Autodesk Fusion 360 part; units mm, degrees
(part 3 of 4)
  line L250 (188.6977, -24.525) -> (178.6977, -24.525)
  arc A251 (178.6977, -21.525) -> (178.6977, -24.525) centre (178.6977, -23.025) ccw
  line L251 (178.6977, -21.525) -> (188.6977, -21.525)
  arc A252 (188.6977, -34.525) -> (188.6977, -31.525) centre (188.6977, -33.025) ccw
  line L252 (188.6977, -34.525) -> (178.6977, -34.525)
  arc A253 (178.6977, -31.525) -> (178.6977, -34.525) centre (178.6977, -33.025) ccw
  line L253 (178.6977, -31.525) -> (188.6977, -31.525)
  arc A254 (88.6977, -34.525) -> (88.6977, -31.525) centre (88.6977, -33.025) ccw
  line L254 (88.6977, -34.525) -> (78.6977, -34.525)
  arc A255 (78.6977, -31.525) -> (78.6977, -34.525) centre (78.6977, -33.025) ccw
  line L255 (78.6977, -31.525) -> (88.6977, -31.525)
  arc A256 (228.6977, -64.525) -> (228.6977, -61.525) centre (228.6977, -63.025) ccw
  line L256 (228.6977, -64.525) -> (218.6977, -64.525)
  arc A257 (218.6977, -61.525) -> (218.6977, -64.525) centre (218.6977, -63.025) ccw
  line L257 (218.6977, -61.525) -> (228.6977, -61.525)
  arc A258 (148.6977, -14.525) -> (148.6977, -11.525) centre (148.6977, -13.025) ccw
  line L258 (148.6977, -14.525) -> (138.6977, -14.525)
  arc A259 (138.6977, -11.525) -> (138.6977, -14.525) centre (138.6977, -13.025) ccw
  line L259 (138.6977, -11.525) -> (148.6977, -11.525)
  arc A260 (208.6977, -54.525) -> (208.6977, -51.525) centre (208.6977, -53.025) ccw
  line L260 (208.6977, -54.525) -> (198.6977, -54.525)
  arc A261 (198.6977, -51.525) -> (198.6977, -54.525) centre (198.6977, -53.025) ccw
  line L261 (198.6977, -51.525) -> (208.6977, -51.525)
  arc A262 (148.6977, -44.525) -> (148.6977, -41.525) centre (148.6977, -43.025) ccw
  line L262 (148.6977, -44.525) -> (138.6977, -44.525)
  arc A263 (138.6977, -41.525) -> (138.6977, -44.525) centre (138.6977, -43.025) ccw
  line L263 (138.6977, -41.525) -> (148.6977, -41.525)
  arc A264 (108.6977, -54.525) -> (108.6977, -51.525) centre (108.6977, -53.025) ccw
  line L264 (108.6977, -54.525) -> (98.6977, -54.525)
  arc A265 (98.6977, -51.525) -> (98.6977, -54.525) centre (98.6977, -53.025) ccw
  line L265 (98.6977, -51.525) -> (108.6977, -51.525)
  arc A266 (108.6977, -24.525) -> (108.6977, -21.525) centre (108.6977, -23.025) ccw
  line L266 (108.6977, -24.525) -> (98.6977, -24.525)
  arc A267 (98.6977, -21.525) -> (98.6977, -24.525) centre (98.6977, -23.025) ccw
  line L267 (98.6977, -21.525) -> (108.6977, -21.525)
  arc A268 (168.6977, -44.525) -> (168.6977, -41.525) centre (168.6977, -43.025) ccw
  line L268 (168.6977, -44.525) -> (158.6977, -44.525)
  arc A269 (158.6977, -41.525) -> (158.6977, -44.525) centre (158.6977, -43.025) ccw
  line L269 (158.6977, -41.525) -> (168.6977, -41.525)
  arc A270 (168.6977, -54.525) -> (168.6977, -51.525) centre (168.6977, -53.025) ccw
  line L270 (168.6977, -54.525) -> (158.6977, -54.525)
  arc A271 (158.6977, -51.525) -> (158.6977, -54.525) centre (158.6977, -53.025) ccw
  line L271 (158.6977, -51.525) -> (168.6977, -51.525)
  arc A272 (148.6977, -34.525) -> (148.6977, -31.525) centre (148.6977, -33.025) ccw
  line L272 (148.6977, -34.525) -> (138.6977, -34.525)
  arc A273 (138.6977, -31.525) -> (138.6977, -34.525) centre (138.6977, -33.025) ccw
  line L273 (138.6977, -31.525) -> (148.6977, -31.525)
  arc A274 (228.6977, -34.525) -> (228.6977, -31.525) centre (228.6977, -33.025) ccw
  line L274 (228.6977, -34.525) -> (218.6977, -34.525)
  arc A275 (218.6977, -31.525) -> (218.6977, -34.525) centre (218.6977, -33.025) ccw
  line L275 (218.6977, -31.525) -> (228.6977, -31.525)
  arc A276 (128.6977, -14.525) -> (128.6977, -11.525) centre (128.6977, -13.025) ccw
  line L276 (128.6977, -14.525) -> (118.6977, -14.525)
  arc A277 (118.6977, -11.525) -> (118.6977, -14.525) centre (118.6977, -13.025) ccw
  line L277 (118.6977, -11.525) -> (128.6977, -11.525)
  arc A278 (108.6977, -44.525) -> (108.6977, -41.525) centre (108.6977, -43.025) ccw
  line L278 (108.6977, -44.525) -> (98.6977, -44.525)
  arc A279 (98.6977, -41.525) -> (98.6977, -44.525) centre (98.6977, -43.025) ccw
  line L279 (98.6977, -41.525) -> (108.6977, -41.525)
  arc A280 (248.6977, -54.525) -> (248.6977, -51.525) centre (248.6977, -53.025) ccw
  line L280 (248.6977, -54.525) -> (238.6977, -54.525)
  arc A281 (238.6977, -51.525) -> (238.6977, -54.525) centre (238.6977, -53.025) ccw
  line L281 (238.6977, -51.525) -> (248.6977, -51.525)
  arc A282 (128.6977, -24.525) -> (128.6977, -21.525) centre (128.6977, -23.025) ccw
  line L282 (128.6977, -24.525) -> (118.6977, -24.525)
  arc A283 (118.6977, -21.525) -> (118.6977, -24.525) centre (118.6977, -23.025) ccw
  line L283 (118.6977, -21.525) -> (128.6977, -21.525)
  arc A284 (108.6977, -34.525) -> (108.6977, -31.525) centre (108.6977, -33.025) ccw
  line L284 (108.6977, -34.525) -> (98.6977, -34.525)
  arc A285 (98.6977, -31.525) -> (98.6977, -34.525) centre (98.6977, -33.025) ccw
  line L285 (98.6977, -31.525) -> (108.6977, -31.525)
  arc A286 (148.6977, -24.525) -> (148.6977, -21.525) centre (148.6977, -23.025) ccw
  line L286 (148.6977, -24.525) -> (138.6977, -24.525)
  arc A287 (138.6977, -21.525) -> (138.6977, -24.525) centre (138.6977, -23.025) ccw
  line L287 (138.6977, -21.525) -> (148.6977, -21.525)
  arc A288 (148.6977, 35.475) -> (148.6977, 38.475) centre (148.6977, 36.975) ccw
  line L288 (148.6977, 35.475) -> (138.6977, 35.475)
  arc A289 (138.6977, 38.475) -> (138.6977, 35.475) centre (138.6977, 36.975) ccw
  line L289 (138.6977, 38.475) -> (148.6977, 38.475)
  arc A290 (208.6977, 15.475) -> (208.6977, 18.475) centre (208.6977, 16.975) ccw
  line L290 (208.6977, 15.475) -> (198.6977, 15.475)
  arc A291 (198.6977, 18.475) -> (198.6977, 15.475) centre (198.6977, 16.975) ccw
  line L291 (198.6977, 18.475) -> (208.6977, 18.475)
  arc A292 (148.6977, 5.475) -> (148.6977, 8.475) centre (148.6977, 6.975) ccw
  line L292 (148.6977, 5.475) -> (138.6977, 5.475)
  arc A293 (138.6977, 8.475) -> (138.6977, 5.475) centre (138.6977, 6.975) ccw
  line L293 (138.6977, 8.475) -> (148.6977, 8.475)
  arc A294 (228.6977, -4.525) -> (228.6977, -1.525) centre (228.6977, -3.025) ccw
  line L294 (228.6977, -4.525) -> (218.6977, -4.525)
  arc A295 (218.6977, -1.525) -> (218.6977, -4.525) centre (218.6977, -3.025) ccw
  line L295 (218.6977, -1.525) -> (228.6977, -1.525)
  arc A296 (188.6977, 15.475) -> (188.6977, 18.475) centre (188.6977, 16.975) ccw
  line L296 (188.6977, 15.475) -> (178.6977, 15.475)
  arc A297 (178.6977, 18.475) -> (178.6977, 15.475) centre (178.6977, 16.975) ccw
  line L297 (178.6977, 18.475) -> (188.6977, 18.475)
  arc A298 (208.6977, -4.525) -> (208.6977, -1.525) centre (208.6977, -3.025) ccw
  line L298 (208.6977, -4.525) -> (198.6977, -4.525)
  arc A299 (198.6977, -1.525) -> (198.6977, -4.525) centre (198.6977, -3.025) ccw
  line L299 (198.6977, -1.525) -> (208.6977, -1.525)
  arc A300 (148.6977, 15.475) -> (148.6977, 18.475) centre (148.6977, 16.975) ccw
  line L300 (148.6977, 15.475) -> (138.6977, 15.475)
  arc A301 (138.6977, 18.475) -> (138.6977, 15.475) centre (138.6977, 16.975) ccw
  line L301 (138.6977, 18.475) -> (148.6977, 18.475)
  arc A302 (188.6977, 25.475) -> (188.6977, 28.475) centre (188.6977, 26.975) ccw
  line L302 (188.6977, 25.475) -> (178.6977, 25.475)
  arc A303 (178.6977, 28.475) -> (178.6977, 25.475) centre (178.6977, 26.975) ccw
  line L303 (178.6977, 28.475) -> (188.6977, 28.475)
  arc A304 (128.6977, 5.475) -> (128.6977, 8.475) centre (128.6977, 6.975) ccw
  line L304 (128.6977, 5.475) -> (118.6977, 5.475)
  arc A305 (118.6977, 8.475) -> (118.6977, 5.475) centre (118.6977, 6.975) ccw
  line L305 (118.6977, 8.475) -> (128.6977, 8.475)
  arc A306 (168.6977, 25.475) -> (168.6977, 28.475) centre (168.6977, 26.975) ccw
  line L306 (168.6977, 25.475) -> (158.6977, 25.475)
  arc A307 (158.6977, 28.475) -> (158.6977, 25.475) centre (158.6977, 26.975) ccw
  line L307 (158.6977, 28.475) -> (168.6977, 28.475)
  arc A308 (168.6977, -4.525) -> (168.6977, -1.525) centre (168.6977, -3.025) ccw
  line L308 (168.6977, -4.525) -> (158.6977, -4.525)
  arc A309 (158.6977, -1.525) -> (158.6977, -4.525) centre (158.6977, -3.025) ccw
  line L309 (158.6977, -1.525) -> (168.6977, -1.525)
  arc A310 (208.6977, 25.475) -> (208.6977, 28.475) centre (208.6977, 26.975) ccw
  line L310 (208.6977, 25.475) -> (198.6977, 25.475)
  arc A311 (198.6977, 28.475) -> (198.6977, 25.475) centre (198.6977, 26.975) ccw
  line L311 (198.6977, 28.475) -> (208.6977, 28.475)
  arc A312 (168.6977, 35.475) -> (168.6977, 38.475) centre (168.6977, 36.975) ccw
  line L312 (168.6977, 35.475) -> (158.6977, 35.475)
  arc A313 (158.6977, 38.475) -> (158.6977, 35.475) centre (158.6977, 36.975) ccw
  line L313 (158.6977, 38.475) -> (168.6977, 38.475)
  arc A314 (228.6977, 15.475) -> (228.6977, 18.475) centre (228.6977, 16.975) ccw
  line L314 (228.6977, 15.475) -> (218.6977, 15.475)
  arc A315 (218.6977, 18.475) -> (218.6977, 15.475) centre (218.6977, 16.975) ccw
  line L315 (218.6977, 18.475) -> (228.6977, 18.475)
  arc A316 (168.6977, 15.475) -> (168.6977, 18.475) centre (168.6977, 16.975) ccw
  line L316 (168.6977, 15.475) -> (158.6977, 15.475)
  arc A317 (158.6977, 18.475) -> (158.6977, 15.475) centre (158.6977, 16.975) ccw
  line L317 (158.6977, 18.475) -> (168.6977, 18.475)
  arc A318 (188.6977, 5.475) -> (188.6977, 8.475) centre (188.6977, 6.975) ccw
  line L318 (188.6977, 5.475) -> (178.6977, 5.475)
  arc A319 (178.6977, 8.475) -> (178.6977, 5.475) centre (178.6977, 6.975) ccw
  line L319 (178.6977, 8.475) -> (188.6977, 8.475)
  arc A320 (148.6977, -4.525) -> (148.6977, -1.525) centre (148.6977, -3.025) ccw
  line L320 (148.6977, -4.525) -> (138.6977, -4.525)
  arc A321 (138.6977, -1.525) -> (138.6977, -4.525) centre (138.6977, -3.025) ccw
  line L321 (138.6977, -1.525) -> (148.6977, -1.525)
  arc A322 (208.6977, 5.475) -> (208.6977, 8.475) centre (208.6977, 6.975) ccw
  line L322 (208.6977, 5.475) -> (198.6977, 5.475)
  arc A323 (198.6977, 8.475) -> (198.6977, 5.475) centre (198.6977, 6.975) ccw
  line L323 (198.6977, 8.475) -> (208.6977, 8.475)
  arc A324 (168.6977, 5.475) -> (168.6977, 8.475) centre (168.6977, 6.975) ccw
  line L324 (168.6977, 5.475) -> (158.6977, 5.475)
  arc A325 (158.6977, 8.475) -> (158.6977, 5.475) centre (158.6977, 6.975) ccw
  line L325 (158.6977, 8.475) -> (168.6977, 8.475)
  arc A326 (228.6977, 5.475) -> (228.6977, 8.475) centre (228.6977, 6.975) ccw
  line L326 (228.6977, 5.475) -> (218.6977, 5.475)
  arc A327 (218.6977, 8.475) -> (218.6977, 5.475) centre (218.6977, 6.975) ccw
  line L327 (218.6977, 8.475) -> (228.6977, 8.475)
  arc A328 (188.6977, -4.525) -> (188.6977, -1.525) centre (188.6977, -3.025) ccw
  line L328 (188.6977, -4.525) -> (178.6977, -4.525)
  arc A329 (178.6977, -1.525) -> (178.6977, -4.525) centre (178.6977, -3.025) ccw
  line L329 (178.6977, -1.525) -> (188.6977, -1.525)
  arc A330 (148.6977, 25.475) -> (148.6977, 28.475) centre (148.6977, 26.975) ccw
  line L330 (148.6977, 25.475) -> (138.6977, 25.475)
  arc A331 (138.6977, 28.475) -> (138.6977, 25.475) centre (138.6977, 26.975) ccw
  line L331 (138.6977, 28.475) -> (148.6977, 28.475)
  arc A332 (188.6977, 35.475) -> (188.6977, 38.475) centre (188.6977, 36.975) ccw
  line L332 (188.6977, 35.475) -> (178.6977, 35.475)
  arc A333 (178.6977, 38.475) -> (178.6977, 35.475) centre (178.6977, 36.975) ccw
  line L333 (178.6977, 38.475) -> (188.6977, 38.475)
  arc A334 (208.6977, 35.475) -> (208.6977, 38.475) centre (208.6977, 36.975) ccw
  line L334 (208.6977, 35.475) -> (198.6977, 35.475)
  arc A335 (198.6977, 38.475) -> (198.6977, 35.475) centre (198.6977, 36.975) ccw
  line L335 (198.6977, 38.475) -> (208.6977, 38.475)
  line L336 (105.9194, -146.05) -> (128.4396, -191.0218)
  line L337 (128.4396, -191.0218) -> (228.4396, -191.0218)
  line L338 (228.4396, -191.0218) -> (250, -146.0218)
  line L339 (250, -146.0218) -> (269.4662, -146.0492)
  line L340 (269.4662, -146.0492) -> (269.5337, -0.009)
  line L341 (269.5337, -0.009) -> (249.9865, 0)
  line L342 (249.9865, 0) -> (228.4396, 44.9718)
  line L343 (228.4396, 44.9718) -> (128.4396, 44.9718)
  line L344 (128.4396, 44.9718) -> (105.9194, 0)
  line L345 (105.9194, 0) -> (90, 0)
  line L346 (90, 0) -> (60, -38.025)
  line L347 (60, -38.025) -> (17.3954, -46.901)
  line L348 (17.3954, -46.901) -> (17.3954, -99.149)
  line L349 (17.3954, -99.149) -> (60, -108.025)
  line L350 (60, -108.025) -> (90, -146.05)
  line L351 (90, -146.05) -> (105.9194, -146.05)
  line L352 (46.3999, -83.0262) -> (46.3999, -63.0262)
  line L353 (46.3999, -63.0262) -> (53.3999, -63.0262)
  line L354 (53.3999, -63.0262) -> (53.3999, -83.0262)
  line L355 (53.3999, -83.0262) -> (46.3999, -83.0262)
copy_body "Body->Comp1" bodies 1 removing the originals makes body 2 in component "Electronics Plate"
sketch "Sketch9" plane through (0, 5, 0) normal (0, 1, 0) x (-1, 0, 0)
  circle A0 centre (260, -3.75) radius 1.5
  circle A1 centre (245, -3.75) radius 1.5
  circle A2 centre (230, -3.75) radius 1.5
  line L0 (250, -73) -> (238, -73) construction
  line L1 (270, -146) -> (220, -146) construction
  line L2 (220, -146) -> (220, -138.5) construction
  line L3 (220, -138.5) -> (270, -138.5) construction
  line L4 (270, -138.5) -> (270, -146) construction
  circle A3 centre (260, -142.25) radius 1.5
  circle A4 centre (245, -142.25) radius 1.5
  circle A5 centre (230, -142.25) radius 1.5
  dimension "d102" = 3
  dimension "d103" = 3
  dimension "d104" = 3
  dimension "d106" = 15
  dimension "d107" = 15
  dimension "d108" = 50
  dimension "d109" = 7.5
  dimension "d110" = 3
  dimension "d111" = 3
  dimension "d112" = 3
  dimension "d113" = 10
  dimension "d114" = 15
  dimension "d115" = 15
  constraint horizontal L0
  constraint horizontal L1
  constraint vertical L2
  constraint horizontal L3
  constraint vertical L4
  measures "d102" diameter of A0
  measures "d103" diameter of A1
  measures "d104" diameter of A2
  measures "d106" distance of A0.centre A1.centre
  measures "d107" distance of A1.centre A2.centre
  measures "d108" distance of L1.start L1.end
  measures "d109" distance of L1.start L3.end
  measures "d110" diameter of A3
  measures "d111" diameter of A4
  measures "d112" diameter of A5
  measures "d113" distance of L4 A3.centre
  measures "d114" distance of A3.centre A4.centre
  measures "d115" distance of A4.centre A5.centre
extrude "Extrude1" cut sketch "Sketch9" against normal blind 40 bodies 2 in component "Electronics Plate"
fillet "Fillet1" radius 30 2 edges at (-90, 2.5, 0) (-90, 2.5, -146.05) on bodies 2 in component "Electronics Plate"
fillet "Fillet2" radius 5 4 edges at (-269.5337, 2.5, -0.009) (-269.4662, 2.5, -146.0492) (-17.3954, 2.5, -46.901) (-17.3954, 2.5, -99.149) on bodies 2 in component "Electronics Plate"
fillet "Fillet3" radius 20 2 edges at (-60, 2.5, -38.025) (-60, 2.5, -108.025) on bodies 2 in component "Electronics Plate"
fillet "Fillet4" radius 17.5 2 edges at (-105.9194, 2.5, 0) (-105.9194, 2.5, -146.05) on bodies 2 in component "Electronics Plate"
fillet "Fillet5" radius 10 4 edges at (-128.4396, 2.5, -191.0218) (-228.4396, 2.5, -191.0218) (-228.4396, 2.5, 44.9718) (-128.4396, 2.5, 44.9718) on bodies 2 in component "Electronics Plate"
sketch "Sketch10" plane through (0, 5, 0) normal (0, 1, 0) x (-1, 0, 0)
sketch "Sketch11" plane through (0, 5, 0) normal (0, 1, 0) x (-1, 0, 0)
  arc A0 (134.6157, 44.9718) -> (125.6742, 39.4494) centre (134.6157, 34.9718) ccw
  line L0 (125.6742, 39.4494) -> (110.2299, 8.6079)
  arc A1 (98.2523, -0.6672) -> (110.2299, 8.6079) centre (94.5822, 16.4437) ccw
  arc A2 (98.2523, -0.6672) -> (80.9916, -11.4182) centre (104.544, -30) ccw
  line L1 (80.9916, -11.4182) -> (64.5039, -32.3163)
  arc A3 (52.8814, -39.508) -> (64.5039, -32.3163) centre (48.8023, -19.9284) ccw
  line L2 (52.8814, -39.508) -> (21.3756, -46.0717)
  arc A4 (21.3756, -46.0717) -> (17.3954, -50.9667) centre (22.3954, -50.9667) ccw
  line L3 (17.3954, -50.9667) -> (17.3954, -95.0833)
  arc A5 (17.3954, -95.0833) -> (21.3756, -99.9783) centre (22.3954, -95.0833) ccw
  line L4 (21.3756, -99.9783) -> (52.8814, -106.542)
  arc A6 (64.5039, -113.7337) -> (52.8814, -106.542) centre (48.8023, -126.1216) ccw
  line L5 (64.5039, -113.7337) -> (80.9916, -134.6318)
  arc A7 (80.9916, -134.6318) -> (98.2523, -145.3828) centre (104.544, -116.05) ccw
  arc A8 (110.2299, -154.6579) -> (98.2523, -145.3828) centre (94.5822, -162.4937) ccw
  line L6 (110.2299, -154.6579) -> (125.6742, -185.4994)
  arc A9 (125.6742, -185.4994) -> (134.6157, -191.0218) centre (134.6157, -181.0218) ccw
  line L7 (134.6157, -191.0218) -> (222.1423, -191.0218)
  arc A10 (222.1423, -191.0218) -> (231.1606, -185.3427) centre (222.1423, -181.0218) ccw
  line L8 (231.1606, -185.3427) -> (250, -146.0218)
  line L9 (250, -146.0218) -> (264.4614, -146.0422)
  arc A11 (264.4614, -146.0422) -> (269.4685, -141.0445) centre (264.4685, -141.0422) ccw
  line L10 (269.4685, -141.0445) -> (269.5314, -5.009)
  arc A12 (269.5314, -5.009) -> (264.5337, -0.0067) centre (264.5314, -5.0067) ccw
  line L11 (264.5337, -0.0067) -> (249.9865, 0)
  line L12 (249.9865, 0) -> (231.1606, 39.2927)
  arc A13 (231.1606, 39.2927) -> (222.1423, 44.9718) centre (222.1423, 34.9718) ccw
  line L13 (222.1423, 44.9718) -> (134.6157, 44.9718)
  arc A14 (228.7157, -4.5249) -> (229.982, -2.2501) centre (230, -3.75) ccw
  arc A15 (228.6977, -4.525) -> (228.7157, -4.5249) centre (228.6977, -3.025) ccw
  line L14 (228.6977, -4.525) -> (218.6977, -4.525)
  arc A16 (218.6977, -1.525) -> (218.6977, -4.525) centre (218.6977, -3.025) ccw
  line L15 (218.6977, -1.525) -> (228.6977, -1.525)
  arc A17 (229.982, -2.2501) -> (228.6977, -1.525) centre (228.6977, -3.025) ccw
  circle A18 centre (260, -3.75) radius 1.5
  circle A19 centre (260, -142.25) radius 1.5
  circle A20 centre (245, -3.75) radius 1.5
  circle A21 centre (245, -142.25) radius 1.5
  arc A22 (208.6977, 15.475) -> (208.6977, 18.475) centre (208.6977, 16.975) ccw
  line L16 (208.6977, 15.475) -> (198.6977, 15.475)
  arc A23 (198.6977, 18.475) -> (198.6977, 15.475) centre (198.6977, 16.975) ccw
  line L17 (198.6977, 18.475) -> (208.6977, 18.475)
  arc A24 (108.6977, -34.525) -> (108.6977, -31.525) centre (108.6977, -33.025) ccw
  line L18 (108.6977, -34.525) -> (98.6977, -34.525)
  arc A25 (98.6977, -31.525) -> (98.6977, -34.525) centre (98.6977, -33.025) ccw
  line L19 (98.6977, -31.525) -> (108.6977, -31.525)
  arc A26 (88.6977, -44.525) -> (88.6977, -41.525) centre (88.6977, -43.025) ccw
  line L20 (88.6977, -44.525) -> (78.6977, -44.525)
  arc A27 (78.6977, -41.525) -> (78.6977, -44.525) centre (78.6977, -43.025) ccw
  line L21 (78.6977, -41.525) -> (88.6977, -41.525)
  arc A28 (168.6977, -34.525) -> (168.6977, -31.525) centre (168.6977, -33.025) ccw
  line L22 (168.6977, -34.525) -> (158.6977, -34.525)
  arc A29 (158.6977, -31.525) -> (158.6977, -34.525) centre (158.6977, -33.025) ccw
  line L23 (158.6977, -31.525) -> (168.6977, -31.525)
  arc A30 (148.6977, -44.525) -> (148.6977, -41.525) centre (148.6977, -43.025) ccw
  line L24 (148.6977, -44.525) -> (138.6977, -44.525)
  arc A31 (138.6977, -41.525) -> (138.6977, -44.525) centre (138.6977, -43.025) ccw
  line L25 (138.6977, -41.525) -> (148.6977, -41.525)
  arc A32 (168.6977, -24.525) -> (168.6977, -21.525) centre (168.6977, -23.025) ccw
  line L26 (168.6977, -24.525) -> (158.6977, -24.525)
  arc A33 (158.6977, -21.525) -> (158.6977, -24.525) centre (158.6977, -23.025) ccw
  line L27 (158.6977, -21.525) -> (168.6977, -21.525)
  arc A34 (228.6977, -34.525) -> (228.6977, -31.525) centre (228.6977, -33.025) ccw
  line L28 (228.6977, -34.525) -> (218.6977, -34.525)
  arc A35 (218.6977, -31.525) -> (218.6977, -34.525) centre (218.6977, -33.025) ccw
  line L29 (218.6977, -31.525) -> (228.6977, -31.525)
  arc A36 (148.6977, -34.525) -> (148.6977, -31.525) centre (148.6977, -33.025) ccw
  line L30 (148.6977, -34.525) -> (138.6977, -34.525)
  arc A37 (138.6977, -31.525) -> (138.6977, -34.525) centre (138.6977, -33.025) ccw
  line L31 (138.6977, -31.525) -> (148.6977, -31.525)
  arc A38 (148.6977, 5.475) -> (148.6977, 8.475) centre (148.6977, 6.975) ccw
  line L32 (148.6977, 5.475) -> (138.6977, 5.475)
  arc A39 (138.6977, 8.475) -> (138.6977, 5.475) centre (138.6977, 6.975) ccw
  line L33 (138.6977, 8.475) -> (148.6977, 8.475)
  arc A40 (168.6977, -4.525) -> (168.6977, -1.525) centre (168.6977, -3.025) ccw
  line L34 (168.6977, -4.525) -> (158.6977, -4.525)
  arc A41 (158.6977, -1.525) -> (158.6977, -4.525) centre (158.6977, -3.025) ccw
  line L35 (158.6977, -1.525) -> (168.6977, -1.525)
  arc A42 (228.6977, -14.525) -> (228.6977, -11.525) centre (228.6977, -13.025) ccw
  line L36 (228.6977, -14.525) -> (218.6977, -14.525)
  arc A43 (218.6977, -11.525) -> (218.6977, -14.525) centre (218.6977, -13.025) ccw
  line L37 (218.6977, -11.525) -> (228.6977, -11.525)
  arc A44 (168.6977, -14.525) -> (168.6977, -11.525) centre (168.6977, -13.025) ccw
  line L38 (168.6977, -14.525) -> (158.6977, -14.525)
  arc A45 (158.6977, -11.525) -> (158.6977, -14.525) centre (158.6977, -13.025) ccw
  line L39 (158.6977, -11.525) -> (168.6977, -11.525)
  arc A46 (188.6977, -34.525) -> (188.6977, -31.525) centre (188.6977, -33.025) ccw
  line L40 (188.6977, -34.525) -> (178.6977, -34.525)
  arc A47 (178.6977, -31.525) -> (178.6977, -34.525) centre (178.6977, -33.025) ccw
  line L41 (178.6977, -31.525) -> (188.6977, -31.525)
  arc A48 (148.6977, -4.525) -> (148.6977, -1.525) centre (148.6977, -3.025) ccw
  line L42 (148.6977, -4.525) -> (138.6977, -4.525)
  arc A49 (138.6977, -1.525) -> (138.6977, -4.525) centre (138.6977, -3.025) ccw
  line L43 (138.6977, -1.525) -> (148.6977, -1.525)
  arc A50 (108.6977, -14.525) -> (108.6977, -11.525) centre (108.6977, -13.025) ccw
  line L44 (108.6977, -14.525) -> (98.6977, -14.525)
  arc A51 (98.6977, -11.525) -> (98.6977, -14.525) centre (98.6977, -13.025) ccw
  line L45 (98.6977, -11.525) -> (108.6977, -11.525)
  arc A52 (248.6977, -24.525) -> (248.6977, -21.525) centre (248.6977, -23.025) ccw
  line L46 (248.6977, -24.525) -> (238.6977, -24.525)
  arc A53 (238.6977, -21.525) -> (238.6977, -24.525) centre (238.6977, -23.025) ccw
  line L47 (238.6977, -21.525) -> (248.6977, -21.525)
  arc A54 (148.6977, 35.475) -> (148.6977, 38.475) centre (148.6977, 36.975) ccw
  line L48 (148.6977, 35.475) -> (138.6977, 35.475)
  arc A55 (138.6977, 38.475) -> (138.6977, 35.475) centre (138.6977, 36.975) ccw
  line L49 (138.6977, 38.475) -> (148.6977, 38.475)
  arc A56 (128.6977, -4.525) -> (128.6977, -1.525) centre (128.6977, -3.025) ccw
  line L50 (128.6977, -4.525) -> (118.6977, -4.525)
  arc A57 (118.6977, -1.525) -> (118.6977, -4.525) centre (118.6977, -3.025) ccw
  line L51 (118.6977, -1.525) -> (128.6977, -1.525)
  arc A58 (168.6977, 35.475) -> (168.6977, 38.475) centre (168.6977, 36.975) ccw
  line L52 (168.6977, 35.475) -> (158.6977, 35.475)
  arc A59 (158.6977, 38.475) -> (158.6977, 35.475) centre (158.6977, 36.975) ccw
  line L53 (158.6977, 38.475) -> (168.6977, 38.475)
  arc A60 (168.6977, -44.525) -> (168.6977, -41.525) centre (168.6977, -43.025) ccw
  line L54 (168.6977, -44.525) -> (158.6977, -44.525)
  arc A61 (158.6977, -41.525) -> (158.6977, -44.525) centre (158.6977, -43.025) ccw
  line L55 (158.6977, -41.525) -> (168.6977, -41.525)
  arc A62 (248.6977, -54.525) -> (248.6977, -51.525) centre (248.6977, -53.025) ccw
  line L56 (248.6977, -54.525) -> (238.6977, -54.525)
  arc A63 (238.6977, -51.525) -> (238.6977, -54.525) centre (238.6977, -53.025) ccw
  line L57 (238.6977, -51.525) -> (248.6977, -51.525)
  arc A64 (128.6977, -24.525) -> (128.6977, -21.525) centre (128.6977, -23.025) ccw
  line L58 (128.6977, -24.525) -> (118.6977, -24.525)
  arc A65 (118.6977, -21.525) -> (118.6977, -24.525) centre (118.6977, -23.025) ccw
  line L59 (118.6977, -21.525) -> (128.6977, -21.525)
  arc A66 (188.6977, -24.525) -> (188.6977, -21.525) centre (188.6977, -23.025) ccw
  line L60 (188.6977, -24.525) -> (178.6977, -24.525)
  arc A67 (178.6977, -21.525) -> (178.6977, -24.525) centre (178.6977, -23.025) ccw
  line L61 (178.6977, -21.525) -> (188.6977, -21.525)
  arc A68 (228.6977, -44.525) -> (228.6977, -41.525) centre (228.6977, -43.025) ccw
  line L62 (228.6977, -44.525) -> (218.6977, -44.525)
  arc A69 (218.6977, -41.525) -> (218.6977, -44.525) centre (218.6977, -43.025) ccw
  line L63 (218.6977, -41.525) -> (228.6977, -41.525)
  arc A70 (188.6977, -44.525) -> (188.6977, -41.525) centre (188.6977, -43.025) ccw
  line L64 (188.6977, -44.525) -> (178.6977, -44.525)
  arc A71 (178.6977, -41.525) -> (178.6977, -44.525) centre (178.6977, -43.025) ccw
  line L65 (178.6977, -41.525) -> (188.6977, -41.525)
  arc A72 (228.6977, 15.475) -> (228.6977, 18.475) centre (228.6977, 16.975) ccw
  line L66 (228.6977, 15.475) -> (218.6977, 15.475)
  arc A73 (218.6977, 18.475) -> (218.6977, 15.475) centre (218.6977, 16.975) ccw
  line L67 (218.6977, 18.475) -> (228.6977, 18.475)
  arc A74 (148.6977, -74.525) -> (148.6977, -71.525) centre (148.6977, -73.025) ccw
  line L68 (148.6977, -74.525) -> (138.6977, -74.525)
  arc A75 (138.6977, -71.525) -> (138.6977, -74.525) centre (138.6977, -73.025) ccw
  line L69 (138.6977, -71.525) -> (148.6977, -71.525)
  arc A76 (228.6977, -24.525) -> (228.6977, -21.525) centre (228.6977, -23.025) ccw
  line L70 (228.6977, -24.525) -> (218.6977, -24.525)
  arc A77 (218.6977, -21.525) -> (218.6977, -24.525) centre (218.6977, -23.025) ccw
  line L71 (218.6977, -21.525) -> (228.6977, -21.525)
  arc A78 (248.6977, -34.525) -> (248.6977, -31.525) centre (248.6977, -33.025) ccw
  line L72 (248.6977, -34.525) -> (238.6977, -34.525)
  arc A79 (238.6977, -31.525) -> (238.6977, -34.525) centre (238.6977, -33.025) ccw
  line L73 (238.6977, -31.525) -> (248.6977, -31.525)
  arc A80 (128.6977, 5.475) -> (128.6977, 8.475) centre (128.6977, 6.975) ccw
  line L74 (128.6977, 5.475) -> (118.6977, 5.475)
  arc A81 (118.6977, 8.475) -> (118.6977, 5.475) centre (118.6977, 6.975) ccw
  line L75 (118.6977, 8.475) -> (128.6977, 8.475)
  arc A82 (228.6977, 5.475) -> (228.6977, 8.475) centre (228.6977, 6.975) ccw
  line L76 (228.6977, 5.475) -> (218.6977, 5.475)
  arc A83 (218.6977, 8.475) -> (218.6977, 5.475) centre (218.6977, 6.975) ccw
  line L77 (218.6977, 8.475) -> (228.6977, 8.475)
  arc A84 (208.6977, 25.475) -> (208.6977, 28.475) centre (208.6977, 26.975) ccw
  line L78 (208.6977, 25.475) -> (198.6977, 25.475)
  arc A85 (198.6977, 28.475) -> (198.6977, 25.475) centre (198.6977, 26.975) ccw
  line L79 (198.6977, 28.475) -> (208.6977, 28.475)
  arc A86 (148.6977, 15.475) -> (148.6977, 18.475) centre (148.6977, 16.975) ccw
  line L80 (148.6977, 15.475) -> (138.6977, 15.475)
  arc A87 (138.6977, 18.475) -> (138.6977, 15.475) centre (138.6977, 16.975) ccw
  line L81 (138.6977, 18.475) -> (148.6977, 18.475)
  arc A88 (108.6977, -44.525) -> (108.6977, -41.525) centre (108.6977, -43.025) ccw
  line L82 (108.6977, -44.525) -> (98.6977, -44.525)
  arc A89 (98.6977, -41.525) -> (98.6977, -44.525) centre (98.6977, -43.025) ccw
  line L83 (98.6977, -41.525) -> (108.6977, -41.525)
  arc A90 (168.6977, 25.475) -> (168.6977, 28.475) centre (168.6977, 26.975) ccw
  line L84 (168.6977, 25.475) -> (158.6977, 25.475)
  arc A91 (158.6977, 28.475) -> (158.6977, 25.475) centre (158.6977, 26.975) ccw
  line L85 (158.6977, 28.475) -> (168.6977, 28.475)
  arc A92 (88.6977, -34.525) -> (88.6977, -31.525) centre (88.6977, -33.025) ccw
  line L86 (88.6977, -34.525) -> (78.6977, -34.525)
  arc A93 (78.6977, -31.525) -> (78.6977, -34.525) centre (78.6977, -33.025) ccw
  line L87 (78.6977, -31.525) -> (88.6977, -31.525)
  arc A94 (208.6977, -44.525) -> (208.6977, -41.525) centre (208.6977, -43.025) ccw
  line L88 (208.6977, -44.525) -> (198.6977, -44.525)
  arc A95 (198.6977, -41.525) -> (198.6977, -44.525) centre (198.6977, -43.025) ccw
  line L89 (198.6977, -41.525) -> (208.6977, -41.525)
  arc A96 (188.6977, 5.475) -> (188.6977, 8.475) centre (188.6977, 6.975) ccw
  line L90 (188.6977, 5.475) -> (178.6977, 5.475)
  arc A97 (178.6977, 8.475) -> (178.6977, 5.475) centre (178.6977, 6.975) ccw
  line L91 (178.6977, 8.475) -> (188.6977, 8.475)
  arc A98 (168.6977, 15.475) -> (168.6977, 18.475) centre (168.6977, 16.975) ccw
  line L92 (168.6977, 15.475) -> (158.6977, 15.475)
  arc A99 (158.6977, 18.475) -> (158.6977, 15.475) centre (158.6977, 16.975) ccw
  line L93 (158.6977, 18.475) -> (168.6977, 18.475)
  arc A100 (108.6977, -24.525) -> (108.6977, -21.525) centre (108.6977, -23.025) ccw
  line L94 (108.6977, -24.525) -> (98.6977, -24.525)
  arc A101 (98.6977, -21.525) -> (98.6977, -24.525) centre (98.6977, -23.025) ccw
  line L95 (98.6977, -21.525) -> (108.6977, -21.525)
  arc A102 (188.6977, 25.475) -> (188.6977, 28.475) centre (188.6977, 26.975) ccw
  line L96 (188.6977, 25.475) -> (178.6977, 25.475)
  arc A103 (178.6977, 28.475) -> (178.6977, 25.475) centre (178.6977, 26.975) ccw
  line L97 (178.6977, 28.475) -> (188.6977, 28.475)
  arc A104 (248.6977, -14.525) -> (248.6977, -11.525) centre (248.6977, -13.025) ccw
  line L98 (248.6977, -14.525) -> (238.6977, -14.525)
  arc A105 (238.6977, -11.525) -> (238.6977, -14.525) centre (238.6977, -13.025) ccw
  line L99 (238.6977, -11.525) -> (248.6977, -11.525)
  arc A106 (188.6977, -4.525) -> (188.6977, -1.525) centre (188.6977, -3.025) ccw
  line L100 (188.6977, -4.525) -> (178.6977, -4.525)
  arc A107 (178.6977, -1.525) -> (178.6977, -4.525) centre (178.6977, -3.025) ccw
  line L101 (178.6977, -1.525) -> (188.6977, -1.525)
  arc A108 (248.6977, -44.525) -> (248.6977, -41.525) centre (248.6977, -43.025) ccw
  line L102 (248.6977, -44.525) -> (238.6977, -44.525)
  arc A109 (238.6977, -41.525) -> (238.6977, -44.525) centre (238.6977, -43.025) ccw
  line L103 (238.6977, -41.525) -> (248.6977, -41.525)
  arc A110 (148.6977, -14.525) -> (148.6977, -11.525) centre (148.6977, -13.025) ccw
  line L104 (148.6977, -14.525) -> (138.6977, -14.525)
  arc A111 (138.6977, -11.525) -> (138.6977, -14.525) centre (138.6977, -13.025) ccw
  line L105 (138.6977, -11.525) -> (148.6977, -11.525)
  arc A112 (208.6977, 5.475) -> (208.6977, 8.475) centre (208.6977, 6.975) ccw
  line L106 (208.6977, 5.475) -> (198.6977, 5.475)
  arc A113 (198.6977, 8.475) -> (198.6977, 5.475) centre (198.6977, 6.975) ccw
  line L107 (198.6977, 8.475) -> (208.6977, 8.475)
  arc A114 (148.6977, 25.475) -> (148.6977, 28.475) centre (148.6977, 26.975) ccw
  line L108 (148.6977, 25.475) -> (138.6977, 25.475)
  arc A115 (138.6977, 28.475) -> (138.6977, 25.475) centre (138.6977, 26.975) ccw
  line L109 (138.6977, 28.475) -> (148.6977, 28.475)
  arc A116 (128.6977, -34.525) -> (128.6977, -31.525) centre (128.6977, -33.025) ccw
  line L110 (128.6977, -34.525) -> (118.6977, -34.525)
  arc A117 (118.6977, -31.525) -> (118.6977, -34.525) centre (118.6977, -33.025) ccw
  line L111 (118.6977, -31.525) -> (128.6977, -31.525)
  arc A118 (208.6977, 35.475) -> (208.6977, 38.475) centre (208.6977, 36.975) ccw
  line L112 (208.6977, 35.475) -> (198.6977, 35.475)
  arc A119 (198.6977, 38.475) -> (198.6977, 35.475) centre (198.6977, 36.975) ccw
  line L113 (198.6977, 38.475) -> (208.6977, 38.475)
  arc A120 (148.6977, -24.525) -> (148.6977, -21.525) centre (148.6977, -23.025) ccw
  line L114 (148.6977, -24.525) -> (138.6977, -24.525)
  arc A121 (138.6977, -21.525) -> (138.6977, -24.525) centre (138.6977, -23.025) ccw
  line L115 (138.6977, -21.525) -> (148.6977, -21.525)
  arc A122 (208.6977, -34.525) -> (208.6977, -31.525) centre (208.6977, -33.025) ccw
  line L116 (208.6977, -34.525) -> (198.6977, -34.525)
  arc A123 (198.6977, -31.525) -> (198.6977, -34.525) centre (198.6977, -33.025) ccw
  line L117 (198.6977, -31.525) -> (208.6977, -31.525)
  arc A124 (128.6977, -44.525) -> (128.6977, -41.525) centre (128.6977, -43.025) ccw
  line L118 (128.6977, -44.525) -> (118.6977, -44.525)
  arc A125 (118.6977, -41.525) -> (118.6977, -44.525) centre (118.6977, -43.025) ccw
  line L119 (118.6977, -41.525) -> (128.6977, -41.525)
  arc A126 (148.6977, -94.525) -> (148.6977, -91.525) centre (148.6977, -93.025) ccw
  line L120 (148.6977, -94.525) -> (138.6977, -94.525)
  arc A127 (138.6977, -91.525) -> (138.6977, -94.525) centre (138.6977, -93.025) ccw
  line L121 (138.6977, -91.525) -> (148.6977, -91.525)
  arc A128 (148.6977, -154.525) -> (148.6977, -151.525) centre (148.6977, -153.025) ccw
  line L122 (148.6977, -154.525) -> (138.6977, -154.525)
  arc A129 (138.6977, -151.525) -> (138.6977, -154.525) centre (138.6977, -153.025) ccw
  line L123 (138.6977, -151.525) -> (148.6977, -151.525)
  arc A130 (148.6977, -104.525) -> (148.6977, -101.525) centre (148.6977, -103.025) ccw
  line L124 (148.6977, -104.525) -> (138.6977, -104.525)
  arc A131 (138.6977, -101.525) -> (138.6977, -104.525) centre (138.6977, -103.025) ccw
  line L125 (138.6977, -101.525) -> (148.6977, -101.525)
  arc A132 (208.6977, -74.525) -> (208.6977, -71.525) centre (208.6977, -73.025) ccw
  line L126 (208.6977, -74.525) -> (198.6977, -74.525)
  arc A133 (198.6977, -71.525) -> (198.6977, -74.525) centre (198.6977, -73.025) ccw
  line L127 (198.6977, -71.525) -> (208.6977, -71.525)
  arc A134 (148.6977, -64.525) -> (148.6977, -61.525) centre (148.6977, -63.025) ccw
  line L128 (148.6977, -64.525) -> (138.6977, -64.525)
  arc A135 (138.6977, -61.525) -> (138.6977, -64.525) centre (138.6977, -63.025) ccw
  line L129 (138.6977, -61.525) -> (148.6977, -61.525)
  arc A136 (168.6977, -124.525) -> (168.6977, -121.525) centre (168.6977, -123.025) ccw
  line L130 (168.6977, -124.525) -> (158.6977, -124.525)
  arc A137 (158.6977, -121.525) -> (158.6977, -124.525) centre (158.6977, -123.025) ccw
  line L131 (158.6977, -121.525) -> (168.6977, -121.525)
  arc A138 (68.6977, -94.525) -> (68.6977, -91.525) centre (68.6977, -93.025) ccw
  line L132 (68.6977, -94.525) -> (58.6977, -94.525)
  arc A139 (58.6977, -91.525) -> (58.6977, -94.525) centre (58.6977, -93.025) ccw
  line L133 (58.6977, -91.525) -> (68.6977, -91.525)
  arc A140 (148.6977, -144.525) -> (148.6977, -141.525) centre (148.6977, -143.025) ccw
  line L134 (148.6977, -144.525) -> (138.6977, -144.525)
  arc A141 (138.6977, -141.525) -> (138.6977, -144.525) centre (138.6977, -143.025) ccw
  line L135 (138.6977, -141.525) -> (148.6977, -141.525)
  arc A142 (188.6977, -114.525) -> (188.6977, -111.525) centre (188.6977, -113.025) ccw
  line L136 (188.6977, -114.525) -> (178.6977, -114.525)
  arc A143 (178.6977, -111.525) -> (178.6977, -114.525) centre (178.6977, -113.025) ccw
  line L137 (178.6977, -111.525) -> (188.6977, -111.525)
  arc A144 (148.6977, -124.525) -> (148.6977, -121.525) centre (148.6977, -123.025) ccw
  line L138 (148.6977, -124.525) -> (138.6977, -124.525)
  arc A145 (138.6977, -121.525) -> (138.6977, -124.525) centre (138.6977, -123.025) ccw
  line L139 (138.6977, -121.525) -> (148.6977, -121.525)
  arc A146 (228.6977, -54.525) -> (228.6977, -51.525) centre (228.6977, -53.025) ccw
  line L140 (228.6977, -54.525) -> (218.6977, -54.525)
  arc A147 (218.6977, -51.525) -> (218.6977, -54.525) centre (218.6977, -53.025) ccw
  line L141 (218.6977, -51.525) -> (228.6977, -51.525)
  arc A148 (128.6977, -74.525) -> (128.6977, -71.525) centre (128.6977, -73.025) ccw
  line L142 (128.6977, -74.525) -> (118.6977, -74.525)
  arc A149 (118.6977, -71.525) -> (118.6977, -74.525) centre (118.6977, -73.025) ccw
  line L143 (118.6977, -71.525) -> (128.6977, -71.525)
  arc A150 (208.6977, -24.525) -> (208.6977, -21.525) centre (208.6977, -23.025) ccw
  line L144 (208.6977, -24.525) -> (198.6977, -24.525)
  arc A151 (198.6977, -21.525) -> (198.6977, -24.525) centre (198.6977, -23.025) ccw
  line L145 (198.6977, -21.525) -> (208.6977, -21.525)
  arc A152 (168.6977, -184.525) -> (168.6977, -181.525) centre (168.6977, -183.025) ccw
  line L146 (168.6977, -184.525) -> (158.6977, -184.525)
  arc A153 (158.6977, -181.525) -> (158.6977, -184.525) centre (158.6977, -183.025) ccw
  line L147 (158.6977, -181.525) -> (168.6977, -181.525)
  arc A154 (248.6977, -74.525) -> (248.6977, -71.525) centre (248.6977, -73.025) ccw
  line L148 (248.6977, -74.525) -> (238.6977, -74.525)
  arc A155 (238.6977, -71.525) -> (238.6977, -74.525) centre (238.6977, -73.025) ccw
  line L149 (238.6977, -71.525) -> (248.6977, -71.525)
  arc A156 (168.6977, -164.525) -> (168.6977, -161.525) centre (168.6977, -163.025) ccw
  line L150 (168.6977, -164.525) -> (158.6977, -164.525)
  arc A157 (158.6977, -161.525) -> (158.6977, -164.525) centre (158.6977, -163.025) ccw
  line L151 (158.6977, -161.525) -> (168.6977, -161.525)
  arc A158 (188.6977, -184.525) -> (188.6977, -181.525) centre (188.6977, -183.025) ccw
  line L152 (188.6977, -184.525) -> (178.6977, -184.525)
  arc A159 (178.6977, -181.525) -> (178.6977, -184.525) centre (178.6977, -183.025) ccw
  line L153 (178.6977, -181.525) -> (188.6977, -181.525)
  arc A160 (208.6977, -114.525) -> (208.6977, -111.525) centre (208.6977, -113.025) ccw
  line L154 (208.6977, -114.525) -> (198.6977, -114.525)
  arc A161 (198.6977, -111.525) -> (198.6977, -114.525) centre (198.6977, -113.025) ccw
  line L155 (198.6977, -111.525) -> (208.6977, -111.525)
  arc A162 (228.6977, -134.525) -> (228.6977, -131.525) centre (228.6977, -133.025) ccw
  line L156 (228.6977, -134.525) -> (218.6977, -134.525)
  arc A163 (218.6977, -131.525) -> (218.6977, -134.525) centre (218.6977, -133.025) ccw
  line L157 (218.6977, -131.525) -> (228.6977, -131.525)
  arc A164 (168.6977, -64.525) -> (168.6977, -61.525) centre (168.6977, -63.025) ccw
  line L158 (168.6977, -64.525) -> (158.6977, -64.525)
  arc A165 (158.6977, -61.525) -> (158.6977, -64.525) centre (158.6977, -63.025) ccw
  line L159 (158.6977, -61.525) -> (168.6977, -61.525)
  arc A166 (208.6977, -94.525) -> (208.6977, -91.525) centre (208.6977, -93.025) ccw
  line L160 (208.6977, -94.525) -> (198.6977, -94.525)
  arc A167 (198.6977, -91.525) -> (198.6977, -94.525) centre (198.6977, -93.025) ccw
  line L161 (198.6977, -91.525) -> (208.6977, -91.525)
  arc A168 (188.6977, -124.525) -> (188.6977, -121.525) centre (188.6977, -123.025) ccw
  line L162 (188.6977, -124.525) -> (178.6977, -124.525)
  arc A169 (178.6977, -121.525) -> (178.6977, -124.525) centre (178.6977, -123.025) ccw
  line L163 (178.6977, -121.525) -> (188.6977, -121.525)
  arc A170 (148.6977, -164.525) -> (148.6977, -161.525) centre (148.6977, -163.025) ccw
  line L164 (148.6977, -164.525) -> (138.6977, -164.525)
  arc A171 (138.6977, -161.525) -> (138.6977, -164.525) centre (138.6977, -163.025) ccw
  line L165 (138.6977, -161.525) -> (148.6977, -161.525)
  arc A172 (108.6977, -54.525) -> (108.6977, -51.525) centre (108.6977, -53.025) ccw
  line L166 (108.6977, -54.525) -> (98.6977, -54.525)
  arc A173 (98.6977, -51.525) -> (98.6977, -54.525) centre (98.6977, -53.025) ccw
  line L167 (98.6977, -51.525) -> (108.6977, -51.525)
  arc A174 (188.6977, -164.525) -> (188.6977, -161.525) centre (188.6977, -163.025) ccw
  line L168 (188.6977, -164.525) -> (178.6977, -164.525)
  arc A175 (178.6977, -161.525) -> (178.6977, -164.525) centre (178.6977, -163.025) ccw
  line L169 (178.6977, -161.525) -> (188.6977, -161.525)
  arc A176 (108.6977, -64.525) -> (108.6977, -61.525) centre (108.6977, -63.025) ccw
  line L170 (108.6977, -64.525) -> (98.6977, -64.525)
  arc A177 (98.6977, -61.525) -> (98.6977, -64.525) centre (98.6977, -63.025) ccw
  line L171 (98.6977, -61.525) -> (108.6977, -61.525)
  arc A178 (108.6977, -84.525) -> (108.6977, -81.525) centre (108.6977, -83.025) ccw
  line L172 (108.6977, -84.525) -> (98.6977, -84.525)
  arc A179 (98.6977, -81.525) -> (98.6977, -84.525) centre (98.6977, -83.025) ccw
  line L173 (98.6977, -81.525) -> (108.6977, -81.525)
  arc A180 (228.6977, -154.525) -> (228.6977, -151.525) centre (228.6977, -153.025) ccw
  line L174 (228.6977, -154.525) -> (218.6977, -154.525)
  arc A181 (218.6977, -151.525) -> (218.6977, -154.525) centre (218.6977, -153.025) ccw
  line L175 (218.6977, -151.525) -> (228.6977, -151.525)
  arc A182 (188.6977, -154.525) -> (188.6977, -151.525) centre (188.6977, -153.025) ccw
  line L176 (188.6977, -154.525) -> (178.6977, -154.525)
  arc A183 (178.6977, -151.525) -> (178.6977, -154.525) centre (178.6977, -153.025) ccw
  line L177 (178.6977, -151.525) -> (188.6977, -151.525)
  arc A184 (108.6977, -74.525) -> (108.6977, -71.525) centre (108.6977, -73.025) ccw
  line L178 (108.6977, -74.525) -> (98.6977, -74.525)
  arc A185 (98.6977, -71.525) -> (98.6977, -74.525) centre (98.6977, -73.025) ccw
  line L179 (98.6977, -71.525) -> (108.6977, -71.525)
  arc A186 (88.6977, -64.525) -> (88.6977, -61.525) centre (88.6977, -63.025) ccw
  line L180 (88.6977, -64.525) -> (78.6977, -64.525)
  arc A187 (78.6977, -61.525) -> (78.6977, -64.525) centre (78.6977, -63.025) ccw
  line L181 (78.6977, -61.525) -> (88.6977, -61.525)
  arc A188 (168.6977, -114.525) -> (168.6977, -111.525) centre (168.6977, -113.025) ccw
  line L182 (168.6977, -114.525) -> (158.6977, -114.525)
  arc A189 (158.6977, -111.525) -> (158.6977, -114.525) centre (158.6977, -113.025) ccw
  line L183 (158.6977, -111.525) -> (168.6977, -111.525)
  arc A190 (228.6977, -94.525) -> (228.6977, -91.525) centre (228.6977, -93.025) ccw
  line L184 (228.6977, -94.525) -> (218.6977, -94.525)
  arc A191 (218.6977, -91.525) -> (218.6977, -94.525) centre (218.6977, -93.025) ccw
  line L185 (218.6977, -91.525) -> (228.6977, -91.525)
  arc A192 (208.6977, -84.525) -> (208.6977, -81.525) centre (208.6977, -83.025) ccw
  line L186 (208.6977, -84.525) -> (198.6977, -84.525)
  arc A193 (198.6977, -81.525) -> (198.6977, -84.525) centre (198.6977, -83.025) ccw
  line L187 (198.6977, -81.525) -> (208.6977, -81.525)
  arc A194 (88.6977, -54.525) -> (88.6977, -51.525) centre (88.6977, -53.025) ccw
  line L188 (88.6977, -54.525) -> (78.6977, -54.525)
  arc A195 (78.6977, -51.525) -> (78.6977, -54.525) centre (78.6977, -53.025) ccw
  line L189 (78.6977, -51.525) -> (88.6977, -51.525)
  arc A196 (188.6977, -14.525) -> (188.6977, -11.525) centre (188.6977, -13.025) ccw
  line L190 (188.6977, -14.525) -> (178.6977, -14.525)
  arc A197 (178.6977, -11.525) -> (178.6977, -14.525) centre (178.6977, -13.025) ccw
  line L191 (178.6977, -11.525) -> (188.6977, -11.525)
  arc A198 (148.6977, -184.525) -> (148.6977, -181.525) centre (148.6977, -183.025) ccw
  line L192 (148.6977, -184.525) -> (138.6977, -184.525)
  arc A199 (138.6977, -181.525) -> (138.6977, -184.525) centre (138.6977, -183.025) ccw
  line L193 (138.6977, -181.525) -> (148.6977, -181.525)
  arc A200 (208.6977, -54.525) -> (208.6977, -51.525) centre (208.6977, -53.025) ccw
  line L194 (208.6977, -54.525) -> (198.6977, -54.525)
  arc A201 (198.6977, -51.525) -> (198.6977, -54.525) centre (198.6977, -53.025) ccw
  line L195 (198.6977, -51.525) -> (208.6977, -51.525)
  arc A202 (68.6977, -54.525) -> (68.6977, -51.525) centre (68.6977, -53.025) ccw
  line L196 (68.6977, -54.525) -> (58.6977, -54.525)
  arc A203 (58.6977, -51.525) -> (58.6977, -54.525) centre (58.6977, -53.025) ccw
  line L197 (58.6977, -51.525) -> (68.6977, -51.525)
  arc A204 (208.6977, -64.525) -> (208.6977, -61.525) centre (208.6977, -63.025) ccw
  line L198 (208.6977, -64.525) -> (198.6977, -64.525)
  arc A205 (198.6977, -61.525) -> (198.6977, -64.525) centre (198.6977, -63.025) ccw
  line L199 (198.6977, -61.525) -> (208.6977, -61.525)
  arc A206 (208.6977, -174.525) -> (208.6977, -171.525) centre (208.6977, -173.025) ccw
  line L200 (208.6977, -174.525) -> (198.6977, -174.525)
  arc A207 (198.6977, -171.525) -> (198.6977, -174.525) centre (198.6977, -173.025) ccw
  line L201 (198.6977, -171.525) -> (208.6977, -171.525)
  arc A208 (168.6977, -144.525) -> (168.6977, -141.525) centre (168.6977, -143.025) ccw
  line L202 (168.6977, -144.525) -> (158.6977, -144.525)
  arc A209 (158.6977, -141.525) -> (158.6977, -144.525) centre (158.6977, -143.025) ccw
  line L203 (158.6977, -141.525) -> (168.6977, -141.525)
  arc A210 (68.6977, -64.525) -> (68.6977, -61.525) centre (68.6977, -63.025) ccw
  line L204 (68.6977, -64.525) -> (58.6977, -64.525)
  arc A211 (58.6977, -61.525) -> (58.6977, -64.525) centre (58.6977, -63.025) ccw
  line L205 (58.6977, -61.525) -> (68.6977, -61.525)
  arc A212 (248.6977, -124.525) -> (248.6977, -121.525) centre (248.6977, -123.025) ccw
  line L206 (248.6977, -124.525) -> (238.6977, -124.525)
  arc A213 (238.6977, -121.525) -> (238.6977, -124.525) centre (238.6977, -123.025) ccw
  line L207 (238.6977, -121.525) -> (248.6977, -121.525)
  arc A214 (228.6977, -124.525) -> (228.6977, -121.525) centre (228.6977, -123.025) ccw
  line L208 (228.6977, -124.525) -> (218.6977, -124.525)
  arc A215 (218.6977, -121.525) -> (218.6977, -124.525) centre (218.6977, -123.025) ccw
  line L209 (218.6977, -121.525) -> (228.6977, -121.525)
  arc A216 (208.6977, -144.525) -> (208.6977, -141.525) centre (208.6977, -143.025) ccw
  line L210 (208.6977, -144.525) -> (198.6977, -144.525)
  arc A217 (198.6977, -141.525) -> (198.6977, -144.525) centre (198.6977, -143.025) ccw
  line L211 (198.6977, -141.525) -> (208.6977, -141.525)
  arc A218 (148.6977, -134.525) -> (148.6977, -131.525) centre (148.6977, -133.025) ccw
  line L212 (148.6977, -134.525) -> (138.6977, -134.525)
  arc A219 (138.6977, -131.525) -> (138.6977, -134.525) centre (138.6977, -133.025) ccw
  line L213 (138.6977, -131.525) -> (148.6977, -131.525)
  arc A220 (188.6977, -64.525) -> (188.6977, -61.525) centre (188.6977, -63.025) ccw
  line L214 (188.6977, -64.525) -> (178.6977, -64.525)
  arc A221 (178.6977, -61.525) -> (178.6977, -64.525) centre (178.6977, -63.025) ccw
  line L215 (178.6977, -61.525) -> (188.6977, -61.525)
  arc A222 (168.6977, -174.525) -> (168.6977, -171.525) centre (168.6977, -173.025) ccw
  line L216 (168.6977, -174.525) -> (158.6977, -174.525)
  arc A223 (158.6977, -171.525) -> (158.6977, -174.525) centre (158.6977, -173.025) ccw
  line L217 (158.6977, -171.525) -> (168.6977, -171.525)
  arc A224 (228.6977, -114.525) -> (228.6977, -111.525) centre (228.6977, -113.025) ccw
  line L218 (228.6977, -114.525) -> (218.6977, -114.525)
  arc A225 (218.6977, -111.525) -> (218.6977, -114.525) centre (218.6977, -113.025) ccw
  line L219 (218.6977, -111.525) -> (228.6977, -111.525)
  arc A226 (128.6977, -94.525) -> (128.6977, -91.525) centre (128.6977, -93.025) ccw
  line L220 (128.6977, -94.525) -> (118.6977, -94.525)
  arc A227 (118.6977, -91.525) -> (118.6977, -94.525) centre (118.6977, -93.025) ccw
  line L221 (118.6977, -91.525) -> (128.6977, -91.525)
  arc A228 (168.6977, 5.475) -> (168.6977, 8.475) centre (168.6977, 6.975) ccw
  line L222 (168.6977, 5.475) -> (158.6977, 5.475)
  arc A229 (158.6977, 8.475) -> (158.6977, 5.475) centre (158.6977, 6.975) ccw
  line L223 (158.6977, 8.475) -> (168.6977, 8.475)
  arc A230 (188.6977, -74.525) -> (188.6977, -71.525) centre (188.6977, -73.025) ccw
  line L224 (188.6977, -74.525) -> (178.6977, -74.525)
  arc A231 (178.6977, -71.525) -> (178.6977, -74.525) centre (178.6977, -73.025) ccw
  line L225 (178.6977, -71.525) -> (188.6977, -71.525)
  arc A232 (108.6977, -114.525) -> (108.6977, -111.525) centre (108.6977, -113.025) ccw
  line L226 (108.6977, -114.525) -> (98.6977, -114.525)
  arc A233 (98.6977, -111.525) -> (98.6977, -114.525) centre (98.6977, -113.025) ccw
  line L227 (98.6977, -111.525) -> (108.6977, -111.525)
  arc A234 (208.6977, -104.525) -> (208.6977, -101.525) centre (208.6977, -103.025) ccw
  line L228 (208.6977, -104.525) -> (198.6977, -104.525)
  arc A235 (198.6977, -101.525) -> (198.6977, -104.525) centre (198.6977, -103.025) ccw
  line L229 (198.6977, -101.525) -> (208.6977, -101.525)
  arc A236 (208.6977, -154.525) -> (208.6977, -151.525) centre (208.6977, -153.025) ccw
  line L230 (208.6977, -154.525) -> (198.6977, -154.525)
  arc A237 (198.6977, -151.525) -> (198.6977, -154.525) centre (198.6977, -153.025) ccw
  line L231 (198.6977, -151.525) -> (208.6977, -151.525)
  arc A238 (168.6977, -104.525) -> (168.6977, -101.525) centre (168.6977, -103.025) ccw
  line L232 (168.6977, -104.525) -> (158.6977, -104.525)
  arc A239 (158.6977, -101.525) -> (158.6977, -104.525) centre (158.6977, -103.025) ccw
  line L233 (158.6977, -101.525) -> (168.6977, -101.525)
  arc A240 (188.6977, -174.525) -> (188.6977, -171.525) centre (188.6977, -173.025) ccw
  line L234 (188.6977, -174.525) -> (178.6977, -174.525)
  arc A241 (178.6977, -171.525) -> (178.6977, -174.525) centre (178.6977, -173.025) ccw
  line L235 (178.6977, -171.525) -> (188.6977, -171.525)
  arc A242 (248.6977, -64.525) -> (248.6977, -61.525) centre (248.6977, -63.025) ccw
  line L236 (248.6977, -64.525) -> (238.6977, -64.525)
  arc A243 (238.6977, -61.525) -> (238.6977, -64.525) centre (238.6977, -63.025) ccw
  line L237 (238.6977, -61.525) -> (248.6977, -61.525)
  arc A244 (128.6977, -84.525) -> (128.6977, -81.525) centre (128.6977, -83.025) ccw
  line L238 (128.6977, -84.525) -> (118.6977, -84.525)
  arc A245 (118.6977, -81.525) -> (118.6977, -84.525) centre (118.6977, -83.025) ccw
  line L239 (118.6977, -81.525) -> (128.6977, -81.525)
  arc A246 (88.6977, -114.525) -> (88.6977, -111.525) centre (88.6977, -113.025) ccw
  line L240 (88.6977, -114.525) -> (78.6977, -114.525)
  arc A247 (78.6977, -111.525) -> (78.6977, -114.525) centre (78.6977, -113.025) ccw
  line L241 (78.6977, -111.525) -> (88.6977, -111.525)
  line L242 (46.3999, -83.0262) -> (46.3999, -63.0262)
  line L243 (46.3999, -63.0262) -> (53.3999, -63.0262)
  line L244 (53.3999, -63.0262) -> (53.3999, -83.0262)
  line L245 (53.3999, -83.0262) -> (46.3999, -83.0262)
  arc A248 (230.0109, -143.75) -> (228.6869, -141.525) centre (230, -142.25) ccw
  arc A249 (228.6977, -144.525) -> (230.0109, -143.75) centre (228.6977, -143.025) ccw
  line L246 (228.6977, -144.525) -> (218.6977, -144.525)
  arc A250 (218.6977, -141.525) -> (218.6977, -144.525) centre (218.6977, -143.025) ccw
  line L247 (218.6977, -141.525) -> (228.6869, -141.525)
  arc A251 (168.6977, -94.525) -> (168.6977, -91.525) centre (168.6977, -93.025) ccw